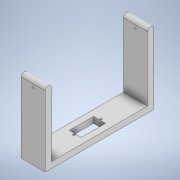
# Autodesk Inventor part: 1st Servo Holder
Saved by Autodesk Inventor 2020.2 (Build 242310000, 310)
## iProperties
Created: 2020-04-02
Part Number: 1st Servo Holder
Material: Generic
Document SubType Name: Modeling
Designer: Amaan Khalid
Density: 1 g/cm^3
Appearance: Default
Author: Amaan Khalid
Autodesk Inventor part; units mm, degrees
ref_plane "YZ Plane" through (0, 0, 0) normal (1, 0, 0) x (0, 1, 0)
ref_plane "XZ Plane" through (0, 0, 0) normal (0, 1, 0) x (-1, 0, 0)
ref_plane "XY Plane" through (0, 0, 0) normal (0, 0, 1) x (1, 0, 0)
sketch "Sketch1" plane through (0, 0, 0) normal (1, 0, 0) x (0, 1, 0)
  point P0 (0, 0)
sketch "Sketch2" plane through (0, 0, 0) normal (1, 0, 0) x (0, 1, 0)
  line L0 (7.3233, 8.5443) -> (7.3233, 8.5443)
  line L1 (4.1483, 5.3693) -> (-70.0914, 5.3693)
  line L2 (4.1483, 11.7193) -> (-63.7414, 11.7193)
  line L3 (-70.0914, 60.6498) -> (-70.0914, 5.3693)
  line L4 (7.3233, 103.7583) -> (7.3233, 103.7583)
  line L5 (-63.7414, 62.4452) -> (-63.7414, 11.7193)
  arc A0 (7.3233, 8.5443) -> (4.1483, 11.7193) centre (4.1483, 8.5443) ccw
  arc A1 (4.1483, 5.3693) -> (7.3233, 8.5443) centre (4.1483, 8.5443) ccw
  line L6 (-70.0914, 60.6498) -> (-70.0914, 119.6333)
  line L7 (-70.0914, 119.6333) -> (4.1483, 119.6333)
  line L8 (-63.7414, 62.4452) -> (-63.7414, 113.2833)
  line L9 (-63.7414, 113.2833) -> (13.8631, 113.2833)
  line L10 (4.1483, 119.6333) -> (4.1483, 119.6333)
  line L11 (7.3233, 116.4583) -> (7.3233, 116.4583)
  arc A2 (7.3233, 116.4583) -> (4.1483, 119.6333) centre (4.1483, 116.4583) ccw
  arc A3 (4.1483, 113.2833) -> (7.3233, 116.4583) centre (4.1483, 116.4583) ccw
  point P0 (0, 0)
  point P1 (7.3233, 11.7193)
  point P2 (7.3233, 5.3693)
  point P3 (7.3233, 106.9333)
  point P4 (7.3233, 100.5833)
  point P5 (7.3233, 8.5443)
  point P6 (7.3233, 119.6333)
  point P7 (4.1483, 113.2833)
  point P8 (4.1483, 119.6333)
  dimension "d0" = 6.35
  dimension "d35" = 3.175
  dimension "d36" = 3.175
  dimension "d42" = 6.35
  dimension "d43" = 6.35
  constraints: 24 end point, 9 point on line, 8 point on circle, 7 tangent, 4 centre point, 3 horizontal, 3 perpendicular, 3 vertical, 2 concentric, 1 horizontal alignment, 3 other
  measures "d0" distance of point (7.323, 11.719) point (7.323, 5.369)
  measures "d35" distance of L7.end point (7.323, 119.633)
  measures "d36" radius of A2
  measures "d42" distance between parallel lines of L8 L6
  measures "d43" distance between parallel lines of L7 L9
extrude "Extrusion1" add sketch "Sketch2" along normal blind 25.4
sketch "Sketch4" plane through (0, -70.0914, 5.3693) normal (0, -1, 0) x (1, 0, 0)
  line L0 (0, 0) -> (25.4, 0) projected
  line L1 (25.4, 114.264) -> (25.4, 0) projected
  line L2 (25.4, 57.132) -> (12.7, 57.132)
  line L3 (19.05, 44.432) -> (6.35, 44.432)
  line L4 (6.35, 44.432) -> (6.35, 69.832)
  line L5 (6.35, 69.832) -> (19.05, 69.832)
  line L6 (19.05, 69.832) -> (19.05, 44.432)
  line L7 (19.05, 44.432) -> (6.35, 69.832) construction
  line L8 (6.35, 44.432) -> (19.05, 69.832) construction
  point P0 (0, -5.3693)
  point P1 (25.4, 101.6762)
  dimension "d48" = 12.7
  dimension "d49" = 25.4
  constraints: 14 end point, 3 midpoint, 2 horizontal, 2 parallel, 1 perpendicular
  measures "d48" distance of L4.end L5.end
  measures "d49" distance of L3.end L4.end
sketch "Sketch6" plane through (0, -70.0914, 119.6333) normal (0, 0, 1) x (1, 0, 0)
  line L0 (0, 77.4147) -> (25.4, 77.4147) projected
  line L1 (0, 77.4147) -> (25.4, 77.4147) projected
  circle A0 centre (12.7, 71.0647) radius 0.9144
  point P0 (0, 70.0914)
  dimension "d45" = 1.8288
  constraints: 1 centre point
  measures "d45" diameter of A0
extrude "Extrusion6" cut sketch "Sketch6" against normal through all
extrude "Extrusion7" cut sketch "Sketch4" against normal through all
sketch "Sketch7" plane through (0, -70.0914, 5.3693) normal (0, -1, 0) x (1, 0, 0)
  line L0 (19.05, 69.832) -> (6.35, 69.832) projected
  line L1 (6.35, 44.432) -> (19.05, 44.432) projected
  circle A0 centre (12.7, 71.356) radius 1.0033
  circle A1 centre (12.7, 42.908) radius 1.0033
  point P0 (0, -5.3693)
  dimension "d55" = 2.0066
  constraints: 2 centre point
  measures "d55" diameter of A1
extrude "Extrusion8" cut sketch "Sketch7" against normal through all
body "Solid1"
